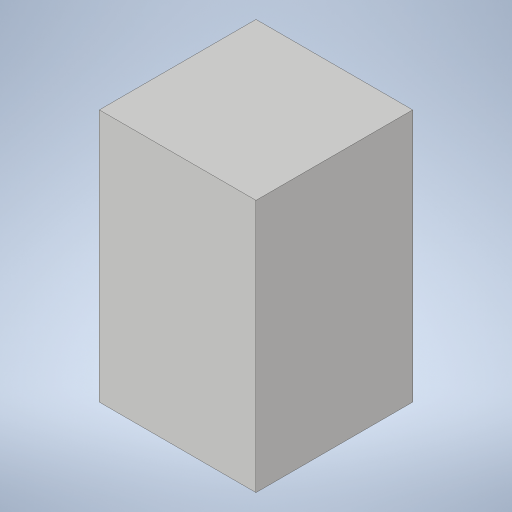
# Autodesk Inventor part: MU-003 Clearance
Saved by Autodesk Inventor 2023.4 (Build 274418000, 418)
## iProperties
Created: 2025-01-05
Part Number: MU-003 Clearance
Material: Generic
Document SubType Name: Modeling
Designer: mavericks
Surface Area: 36903.2 cm^2
Volume: 465262 cm^3
Appearance: Default
Author: mavericks
Autodesk Inventor part; units mm, degrees
ref_plane "YZ Plane" through (0, 0, 0) normal (1, 0, 0) x (0, 1, 0)
ref_plane "XZ Plane" through (0, 0, 0) normal (0, 1, 0) x (-1, 0, 0)
ref_plane "XY Plane" through (0, 0, 0) normal (0, 0, 1) x (1, 0, 0)
sketch "Sketch1" plane through (0, 0, 0) normal (0, 0, 1) x (1, 0, 0)
  line L0 (0, 0) -> (660.4, 0)
  line L1 (660.4, 0) -> (660.4, 1066.8)
  line L2 (660.4, 1066.8) -> (0, 1066.8)
  line L3 (0, 1066.8) -> (0, 0)
  dimension "d0" = 660.4
  dimension "d1" = 1066.8
  constraints: 8 end point, 2 parallel, 1 horizontal, 1 perpendicular
  measures "d0" distance of L2.end L1.end
  measures "d1" distance of L1.end L0.end
extrude "Extrusion1" add sketch "Sketch1" along normal blind 660.4
body "Solid1"
